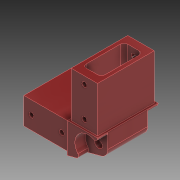
# Autodesk Inventor part: F4C9-200-003 Bottom Bearing Block
Saved by Autodesk Inventor 2021 (Build 250183000, 183)
## iProperties
Created: 2020-08-09
Part Number: F4C9-200-003 Bottom Bearing Block
Material: Aluminum 6061
Document SubType Name: Modeling
Density: 2.7 g/cm^3
Appearance: Reflective - Red
ItemSpecifications: {"_id":"606dcd45c65f90000973f6de","finish":"543ef1f380da5b0c476373c1","finish_location":null,"material":"5515e170db035c20ce34af9a","process_initialism":null,"quotes":null,"current_quote":null,"quantity_ordered":5,"features":null,"hardware":null,"threading":null,"part_markings":[],"surface_roughness":null,"tolerance":null,"weld_quantity":null,"Notes":"","certifications":[],"part":null,"revision_num":0,"last_history":null,"inspection_requirement_details":{"inspection_requirement":"std","customer_data_sheet":null},"feedback":null}
Autodesk Inventor part; units mm, degrees
ref_plane "YZ Plane" through (0, 0, 0) normal (1, 0, 0) x (0, 1, 0)
ref_plane "XZ Plane" through (0, 0, 0) normal (0, 1, 0) x (-1, 0, 0)
ref_plane "XY Plane" through (0, 0, 0) normal (0, 0, 1) x (1, 0, 0)
sketch "Sketch1" plane through (0, 0, 0) normal (0, 0, 1) x (1, 0, 0)
  line L0 (9.525, 38.1) -> (34.925, 38.1) construction
  line L1 (34.925, 38.1) -> (34.925, -12.7) construction
  line L2 (34.925, -12.7) -> (9.525, -12.7) construction
  line L3 (9.525, -12.7) -> (9.525, 38.1) construction
  line L4 (34.925, -12.7) -> (-35.0685, -12.7) construction
  line L5 (-35.0685, -12.7) -> (-35.0685, -38.1) construction
  line L6 (-35.0685, -38.1) -> (34.925, -38.1) construction
  line L7 (34.925, -38.1) -> (34.925, -12.7) construction
  circle A0 centre (0, 0) radius 9.525 construction
  line L8 (7.9375, 50.8) -> (-17.4625, 50.8)
  line L9 (-17.4625, 50.8) -> (-17.4625, 12.7)
  line L10 (-17.4625, 12.7) -> (7.9375, 12.7)
  line L11 (7.9375, 12.7) -> (7.9375, 50.8)
  line L12 (-55.5625, 12.7) -> (-17.4625, 12.7)
  line L13 (-17.4625, 12.7) -> (-17.4625, -12.7)
  line L14 (-17.4625, -12.7) -> (-55.5625, -12.7)
  line L15 (-55.5625, -12.7) -> (-55.5625, 12.7)
  circle A1 centre (0, 0) radius 1.27
  circle A2 centre (0, 0) radius 7.9375
  line L16 (7.9375, 12.7) -> (7.9375, 0)
  line L17 (1.9819, -7.6861) -> (-17.4625, -12.7)
  circle A3 centre (-4.7625, 19.05) radius 2.0193
  circle A4 centre (-4.7625, 44.45) radius 2.0193
  circle A5 centre (-23.8125, 0) radius 2.0193
  circle A6 centre (-49.2125, 0) radius 2.0193
  circle A7 centre (0, 0) radius 11.1125
  point P0 (-4.7625, 50.8)
  point P1 (-55.5625, 0)
  dimension "d0" = 25.4
  dimension "d1" = 50.8
  dimension "d2" = 19.05
  dimension "d3" = 25.4
  dimension "d4" = 3.175
  dimension "d5" = 1.5875
  dimension "d6" = 2.54
  dimension "d7" = 15.875
  dimension "d8" = 38.1
  dimension "d9" = 38.1
  dimension "d10" = 4.0386
  dimension "d13" = 25.4
  dimension "d20" = 25.4
  dimension "d25" = 6.35
  dimension "d26" = 6.35
  dimension "d44" = 1.5875
  constraints: 36 end point, 8 centre point, 8 parallel, 6 perpendicular, 5 horizontal, 3 tangent, 2 coincident, 2 midpoint, 2 point on circle, 1 collinear, 1 equal radius, 1 horizontal alignment, 1 vertical, 1 vertical alignment, 4 other
  measures "d0" distance of L1.end L2.end
  measures "d1" distance of L0.end L1.end
  measures "d2" diameter of A0
  measures "d3" distance of L10.end L9.end
  measures "d4" distance edge to line of A0 L4
  measures "d5" distance between parallel lines of L3 L11
  measures "d6" diameter of A1
  measures "d7" diameter of A2
  measures "d8" distance between parallel lines of L13 L15
  measures "d9" distance between parallel lines of L10 L8
  measures "d10" diameter of A3
  measures "d13" distance of A3.centre A4.centre
  measures "d20" distance of A5.centre A6.centre
  measures "d25" distance from line of L13 A5.centre
  measures "d26" distance from line of L10 A3.centre
  measures "d44" radial gap between concentric circles of A0 A7
extrude "Extrusion1" add sketch "Sketch1" along normal mid plane 50.8 contours L11 L10 L9 L8 | L16 A7 L17 L13 L10 | L13 L14 L15 L12 | L16 A2 L17 A7 | A2 | A1 picked at (-8.4087, 5.384)
sketch "Sketch2" plane through (-17.4625, 50.8, 25.4) normal (0, 1, 0) x (1, 0, 0)
  line L0 (0, 50.8) -> (0, 0) projected
  line L1 (25.4, 0) -> (0, 0) projected
  line L2 (25.4, 50.8) -> (25.4, 0) projected
  line L3 (0, 50.8) -> (25.4, 50.8) projected
  line L4 (1.5875, 1.5875) -> (1.5875, 49.2125)
  line L5 (1.5875, 49.2125) -> (23.8125, 49.2125)
  line L6 (23.8125, 49.2125) -> (23.8125, 1.5875)
  line L7 (23.8125, 1.5875) -> (1.5875, 1.5875)
  line L8 (4.7625, 42.8625) -> (20.6375, 42.8625)
  line L9 (20.6375, 42.8625) -> (20.6375, 7.9375)
  line L10 (20.6375, 7.9375) -> (4.7625, 7.9375)
  line L11 (4.7625, 7.9375) -> (4.7625, 42.8625)
  point P0 (17.4625, 25.4)
  dimension "d29" = 1.5875
  dimension "d40" = 6.35
  dimension "d41" = 6.35
  dimension "d42" = 3.175
  dimension "d43" = 3.175
  constraints: 16 end point, 2 parallel, 1 horizontal, 1 perpendicular, 3 other
  measures "d29" distance between parallel lines of L0 L4
  measures "d40" distance between parallel lines of L7 L10
  measures "d41" distance between parallel lines of L5 L8
  measures "d42" distance between parallel lines of L6 L9
  measures "d43" distance between parallel lines of L4 L11
extrude "Extrusion2" cut sketch "Sketch2" against normal up to surface (38.1 mm away)
sketch "Sketch3" plane through (-55.5625, -12.7, 25.4) normal (-1, 0, 0) x (0, 0, 1)
  line L0 (-50.8, 0) -> (0, 0) projected
  line L1 (0, 25.4) -> (0, 0) projected
  line L2 (0, 25.4) -> (-50.8, 25.4) projected
  line L3 (-50.8, 0) -> (-50.8, 25.4) projected
  line L4 (-49.2125, 23.8125) -> (-1.5875, 23.8125)
  line L5 (-1.5875, 23.8125) -> (-1.5875, 1.5875)
  line L6 (-1.5875, 1.5875) -> (-49.2125, 1.5875)
  line L7 (-49.2125, 1.5875) -> (-49.2125, 23.8125)
  line L8 (-42.8625, 20.6375) -> (-7.9375, 20.6375)
  line L9 (-7.9375, 20.6375) -> (-7.9375, 4.7625)
  line L10 (-7.9375, 4.7625) -> (-42.8625, 4.7625)
  line L11 (-42.8625, 4.7625) -> (-42.8625, 20.6375)
  point P0 (-25.4, 12.7)
  dimension "d32" = 1.5875
  dimension "d35" = 6.35
  dimension "d36" = 6.35
  dimension "d37" = 3.175
  dimension "d38" = 3.175
  constraints: 16 end point, 2 parallel, 1 horizontal, 1 perpendicular, 3 other
  measures "d32" distance between parallel lines of L2 L4
  measures "d35" distance between parallel lines of L5 L9
  measures "d36" distance between parallel lines of L7 L11
  measures "d37" distance between parallel lines of L4 L8
  measures "d38" distance between parallel lines of L6 L10
extrude "Extrusion3" cut sketch "Sketch3" against normal blind 38.1
extrude "Extrusion4" cut sketch "Sketch1" against normal blind 8.7249 from surface at 25.4 contours A7 L17 A2 L16 | L16 A2 L17 A7 | A2 | A1
sketch "Sketch4" plane through (7.9375, 0, 16.6751) normal (0, 0, 1) x (1, 0, 0)
  arc A0 (-5.9556, -7.6861) -> (0, 0) centre (-7.9375, 0) ccw projected
  point P0 (-7.9375, 0)
  constraints: 1 coincident
hole "Hole2" at (0, 0, 16.6751) direction (0, 0, -1) diameter 3.683 depth 13.2842 counterbore diameter 6.35 counterbore depth 3.9624 thread size "10-24 UNC" class "2B" standard "ANSI Unified Screw Threads"
mirror "Mirror1" about plane through (0, 0, 0) normal (0, 0, 1) of "Extrusion4", "Hole2"
fillet "Fillet1" radius 3.175 8 edges at (-36.5125, 7.9375, -17.4625) (-36.5125, 7.9375, 17.4625) (-36.5125, -7.9375, 17.4625) (-36.5125, -7.9375, -17.4625) (3.175, 31.75, 17.4625) (-12.7, 31.75, 17.4625) (-12.7, 31.75, -17.4625) (3.175, 31.75, -17.4625)
fillet "Fillet1" radius 2.286 4 edges at (-5.5489, -9.628, 21.0375) (7.9375, 7.7771, 21.0375) (7.9375, 7.7771, -21.0375) (-5.5489, -9.628, -21.0375)
equation "\"d9\" = d8"
equation "\"d26\" = d25"
equation "\"d41\" = d40"
equation "\"d36\" = d35"
body "Solid1"
